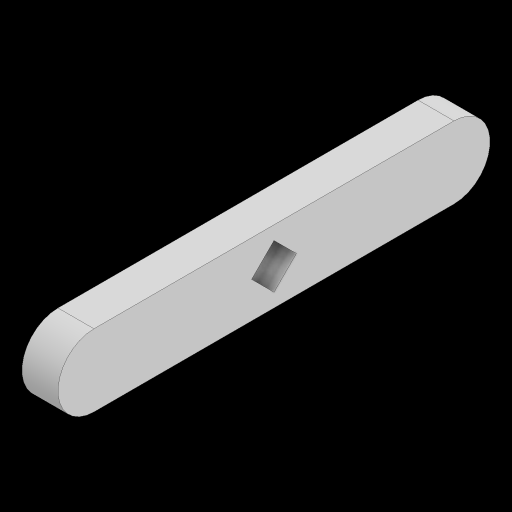
# Autodesk Inventor part: lever_handle
Saved by Autodesk Inventor 2023 (Build 270158000, 158)
## iProperties
Created: 2024-07-10
Part Number: lever_handle
Material: 일반
Document SubType Name: Modeling
Designer: OMS55
Density: 1 g/cm^3
Appearance: 기본값
Author: OMS55
Autodesk Inventor part; units mm, degrees
ref_plane "YZ Plane" through (0, 0, 0) normal (1, 0, 0) x (0, 1, 0)
ref_plane "XZ Plane" through (0, 0, 0) normal (0, 1, 0) x (-1, 0, 0)
ref_plane "XY Plane" through (0, 0, 0) normal (0, 0, 1) x (1, 0, 0)
sketch "스케치1" plane through (0, 0, 0) normal (1, 0, 0) x (0, 1, 0)
  line L0 (0, 25) -> (0, -25) construction
  line L1 (-5, 25) -> (-5, -25)
  line L2 (5, -25) -> (5, 25)
  arc A0 (5, 25) -> (-5, 25) centre (0, 25) ccw
  arc A1 (-5, -25) -> (5, -25) centre (0, -25) ccw
  line L3 (0, 3.1113) -> (-3.1113, 0)
  line L4 (-3.1113, 0) -> (0, -3.1113)
  line L5 (0, -3.1113) -> (3.1113, 0)
  line L6 (3.1113, 0) -> (0, 3.1113)
  point P0 (0, 0)
  point P1 (0, 0)
  dimension "d0" = 50
  dimension "d1" = 5
  dimension "d2" = 4.4
  constraints: 16 end point, 4 point on circle, 4 tangent, 3 parallel, 2 centre point, 2 horizontal alignment, 2 vertical alignment, 1 coincident, 1 midpoint, 1 perpendicular, 1 point on line, 1 vertical
  measures "d0" distance of L2.start L2.end
  measures "d1" radius of A1
  measures "d2" distance of L3.start L3.end
extrude "돌출1" add sketch "스케치1" along normal blind 5
